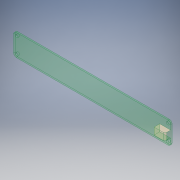
# Autodesk Inventor part: SH8_003.1-sunhub8-PCB
Saved by Autodesk Inventor 2019 (Build 230136000, 136)
## iProperties
Created: 2019-02-22
Part Number: SH8_003.1-sunhub8-PCB
Material: Generic
Document SubType Name: Modeling
Designer: Rene
Density: 1 g/cm^3
Appearance: Clear - Green 1
Author: Rene
Autodesk Inventor part; units mm, degrees
ref_plane "YZ Plane" through (0, 0, 0) normal (1, 0, 0) x (0, 1, 0)
ref_plane "XZ Plane" through (0, 0, 0) normal (0, 1, 0) x (-1, 0, 0)
ref_plane "XY Plane" through (0, 0, 0) normal (0, 0, 1) x (1, 0, 0)
sketch "Sketch1" plane through (0, 0, 0) normal (0, 0, 1) x (1, 0, 0)
  line L0 (-90, -12.5) -> (90, -12.5)
  line L1 (90, -12.5) -> (90, 12.5)
  line L2 (90, 12.5) -> (-90, 12.5)
  line L3 (-90, 12.5) -> (-90, -12.5)
  point P0 (0, 0)
  dimension "d0" = 25
  dimension "d1" = 12.5
  dimension "d2" = 180
  dimension "d3" = 90
  constraints: 8 end point, 2 parallel, 1 horizontal, 1 perpendicular
  measures "d0" distance of L2.end L0.start
  measures "d1" vertical distance of point (0, 0) L0.start
  measures "d2" distance of L0.start L0.end
  measures "d3" horizontal distance of point (0, 0) L0.start
extrude "Extrusion1" add sketch "Sketch1" along normal blind 1.6
fillet "Fillet1" radius 3 4 edges at (-90, -12.5, 0.8) (-90, 12.5, 0.8) (90, -12.5, 0.8) (90, 12.5, 0.8)
sketch "Sketch2" plane through (0, 0, 1.6) normal (0, 0, 1) x (1, 0, 0)
  line L0 (-86.5, 9) -> (86.5, 9) construction
  line L1 (86.5, 9) -> (86.5, -9) construction
  line L2 (86.5, -9) -> (-86.5, -9) construction
  line L3 (-86.5, -9) -> (-86.5, 9) construction
  point P0 (0, 0)
  dimension "d7" = 18
  dimension "d8" = 9
  dimension "d9" = 173
  dimension "d10" = 86.5
  constraints: 8 end point, 4 coincident, 2 parallel, 1 horizontal, 1 perpendicular
  measures "d7" distance of L2.end L0.start
  measures "d8" vertical distance of point (0, 0) L2.end
  measures "d9" distance of L1.end L2.end
  measures "d10" horizontal distance of point (0, 0) L2.end
hole "Hole1" at (-86.5, 9, 1.6) at (-86.5, -9, 1.6) at (86.5, -9, 1.6) at (86.5, 9, 1.6) direction (0, 0, -1) diameter 3.2 end through all
sketch "Sketch4" plane through (0, 0, 1.6) normal (0, 0, 1) x (1, 0, 0)
  line L0 (90, -9.5) -> (90, 9.5) projected
  line L1 (90, 4) -> (77.5, 4)
  line L2 (77.5, 4) -> (77.5, -4)
  line L3 (77.5, -4) -> (90, -4)
  line L4 (90, -4) -> (90, 4)
  point P0 (0, 0)
  dimension "d20" = 8
  dimension "d21" = 4
  dimension "d22" = 12.5
  constraints: 8 end point, 2 parallel, 1 horizontal, 1 perpendicular, 1 point on line
  measures "d20" distance of L1.end L2.end
  measures "d21" vertical distance of point (0, 0) L2.end
  measures "d22" distance of L2.end L3.end
extrude "Extrusion3" add sketch "Sketch4" along normal blind 6.5
chamfer "Chamfer1" distance 2 angle 45 1 edges at (90, 0, 8.1)
equation "\"d1\" = 0.5 * d0"
equation "\"d3\" = 0.5 * d2"
equation "\"d8\" = 0.5 * d7"
equation "\"d10\" = 0.5 * d9"
equation "\"d21\" = 0.5 * d20"
body "Solid1"
